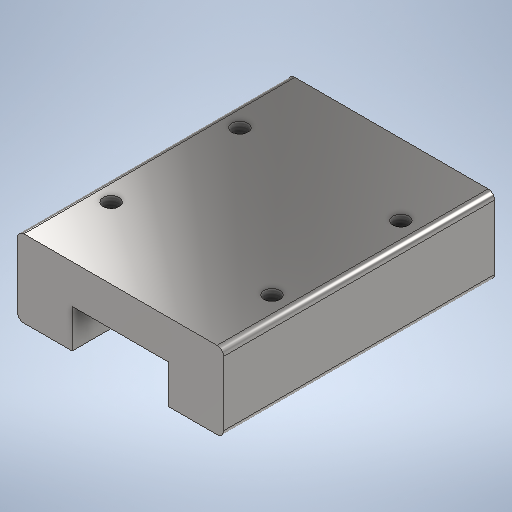
# Autodesk Inventor part: MGN12C Cart
Saved by Autodesk Inventor 2026.2 (Build 302298010, 298A)
## iProperties
Created: 2026-04-28
Part Number: MGN12C Cart
Material: Steel, Carbon
Document SubType Name: Modeling
Designer: chanh
Density: 7.85 g/cm^3
Appearance: Semi-Polished
Author: chanh
Autodesk Inventor part; units mm, degrees
ref_plane "YZ Plane" through (0, 0, 0) normal (1, 0, 0) x (0, 1, 0)
ref_plane "XZ Plane" through (0, 0, 0) normal (0, 1, 0) x (-1, 0, 0)
ref_plane "XY Plane" through (0, 0, 0) normal (0, 0, 1) x (1, 0, 0)
sketch "Sketch1" plane through (0, 0, 0) normal (0, 0, 1) x (1, 0, 0)
  line L0 (-7.5, 6) -> (7.5, 6)
  line L1 (7.5, 6) -> (7.5, 0)
  line L2 (7.5, 0) -> (-7.5, 0)
  line L3 (-7.5, 0) -> (-7.5, 6)
  line L4 (-7.5, 6) -> (7.5, 0) construction
  line L5 (7.5, 6) -> (-7.5, 0) construction
  line L6 (-16, 12) -> (16, 12)
  line L7 (16, 12) -> (16, 0)
  line L8 (16, 0) -> (-16, 0)
  line L9 (-16, 0) -> (-16, 12)
  line L10 (-16, 12) -> (16, 0) construction
  line L11 (16, 12) -> (-16, 0) construction
  point P0 (0, 0)
  point P1 (0, 3)
  point P2 (0, 0)
  point P3 (0, 6)
  point P4 (7.5, 0)
  point P5 (-7.5, 0)
  dimension "d0" = 15
  dimension "d1" = 6
  dimension "d2" = 32
  dimension "d3" = 12
  constraints: 24 end point, 6 midpoint, 4 parallel, 2 horizontal, 2 perpendicular, 1 coincident
  measures "d0" distance of L0.start L0.end
  measures "d1" distance of L0.end L1.end
  measures "d2" distance of L7.end L8.end
  measures "d3" distance of L6.end L7.end
extrude "Extrusion1" add sketch "Sketch1" along normal mid plane 42.1 contours L3 L8 L9 L6 L7 L1 L0
sketch "Sketch2" plane through (-16, 12, 21.05) normal (0, 1, 0) x (1, 0, 0)
  line L0 (28.5, 11.05) -> (3.5, 11.05) construction
  line L1 (3.5, 11.05) -> (3.5, 31.05) construction
  line L2 (3.5, 31.05) -> (28.5, 31.05) construction
  line L3 (28.5, 31.05) -> (28.5, 11.05) construction
  line L4 (28.5, 11.05) -> (3.5, 31.05) construction
  line L5 (3.5, 11.05) -> (28.5, 31.05) construction
  point P0 (16, 21.05)
  dimension "d6" = 25
  dimension "d7" = 20
  constraints: 12 end point, 4 coincident, 2 midpoint, 2 parallel, 1 horizontal, 1 perpendicular
  measures "d6" distance of L1.end L2.end
  measures "d7" distance of L0.end L1.end
hole "Hole1" at (-12.5, 12, 10) at (12.5, 12, 10) at (12.5, 12, -10) at (-12.5, 12, -10) direction (0, -1, 0) diameter 2.459 depth 4 thread size "M3x0.5" class "6H" standard "ISO Metric profile"
fillet "Fillet1" radius 1 4 edges at (16, 12, 0) (-16, 12, 0) (16, 0, 0) (-16, 0, 0)
body "Solid1"
